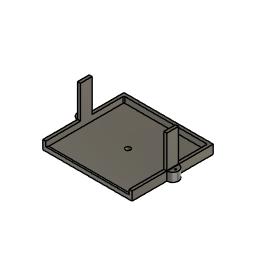
battery tray v7 (Autodesk Fusion 360 design; units mm, degrees)
Autodesk Fusion 360 part; units mm, degrees
sketch "Sketch1" plane through (0, 0, 0) normal (0, 0, 1) x (1, 0, 0)
  line L0 (0, 0) -> (0, 176.2125)
  line L1 (0, 176.2125) -> (193.675, 176.2125)
  line L2 (193.675, 176.2125) -> (193.675, 0)
  line L3 (193.675, 0) -> (0, 0)
  dimension "d21" = 193.675
  dimension "d22" = 176.2125
  constraint coincident L0.start L3.end
  constraint vertical L0
  constraint perpendicular L0 L1
  constraint perpendicular L1 L2
  constraint perpendicular L0 L3
  measures "d21" distance of L0 L2
  measures "d22" distance of L1 L3
extrude "Extrude1" add sketch "Sketch1" along normal blind 19.05
sketch "Sketch3" plane through (0, 0, 19.05) normal (0, 0, 1) x (-1, 0, 0)
  line L0 (-193.675, 0) -> (-193.675, -176.2125)
  line L1 (-193.675, -176.2125) -> (0, -176.2125)
  line L2 (0, -176.2125) -> (0, 0)
  line L3 (0, 0) -> (-193.675, 0)
  line L4 (-187.325, -6.35) -> (-6.35, -6.35)
  line L5 (-6.35, -6.35) -> (-6.35, -167.8305)
  line L6 (-8.382, -169.8625) -> (-185.293, -169.8625)
  line L7 (-187.325, -167.8305) -> (-187.325, -6.35)
  arc A0 (-187.325, -167.8305) -> (-185.293, -169.8625) centre (-185.293, -167.8305) ccw
  arc A1 (-8.382, -169.8625) -> (-6.35, -167.8305) centre (-8.382, -167.8305) ccw
  dimension "d13" = 180.975
  dimension "d14" = 163.5125
  dimension "d17" = 6.35
  dimension "d18" = 6.35
  dimension "d25" = 2.032
  dimension "d26" = 2.032
  constraint horizontal L4
  constraint vertical L5
  constraint horizontal L6
  constraint vertical L7
  constraint tangent L7 A0
  constraint tangent L6 A0
  constraint tangent L5 A1
  constraint tangent L6 A1
  constraint coincident L4.start L7.end
  constraint coincident L4.end L5.start
  measures "d13" distance of L5 L7
  measures "d14" distance of L4 L6
  measures "d17" distance of L3 L4
  measures "d18" distance of L2 L5
  measures "d25" radius of A0
  measures "d26" radius of A1
extrude "Extrude3" cut sketch "Sketch3" against normal blind 12.7 contours L4 L5 L6 L7 A0 A1
sketch "Sketch4" plane through (0, 0, 0) normal (0, 0, 1) x (1, 0, 0)
  line L0 (193.675, 176.2125) -> (193.675, 0)
  circle A0 centre (193.675, 88.1062) radius 12.7
  line L1 (193.675, 0) -> (0, 0)
  line L2 (0, 176.2125) -> (193.675, 176.2125)
  line L3 (0, 0) -> (0, 176.2125)
  circle A1 centre (0, 88.1062) radius 12.7
  dimension "d29" = 88.1063
  dimension "d30" = 88.1063
  dimension "d31" = 25.4
  dimension "d61" = 25.4
  constraint coincident L0 A0.centre
  measures "d29" distance of A0.centre L1
  measures "d30" distance of A0.centre L2
  measures "d31" diameter of A0
  measures "d61" diameter of A1
extrude "Extrude4" add sketch "Sketch4" along normal blind 19.05 contours L0 A0 | L3 A1 picked at (197.7369, 89.2989) picked at (-6.9833, 85.4668)
sketch "Sketch5" plane through (0, 0, 19.05) normal (0, 0, 1) x (-1, 0, 0)
  line L0 (-8.382, -169.8625) -> (-185.293, -169.8625)
  arc A0 (-187.325, -167.8305) -> (-185.293, -169.8625) centre (-185.293, -167.8305) ccw
  line L1 (-187.325, -167.8305) -> (-187.325, -6.35)
  line L2 (-187.325, -6.35) -> (-6.35, -6.35)
  line L3 (-6.35, -6.35) -> (-6.35, -167.8305)
  arc A1 (-8.382, -169.8625) -> (-6.35, -167.8305) centre (-8.382, -167.8305) ccw
  line L4 (-193.675, 0) -> (-193.675, -75.4062)
  arc A2 (-193.675, -75.4062) -> (-193.675, -100.8062) centre (-193.675, -88.1062) ccw
  line L5 (-193.675, -100.8062) -> (-193.675, -176.2125)
  line L6 (-193.675, -176.2125) -> (0, -176.2125)
  line L7 (0, -176.2125) -> (0, -100.8062)
  arc A3 (0, -100.8062) -> (0, -75.4062) centre (0, -88.1062) ccw
  line L8 (0, -75.4062) -> (0, 0)
  line L9 (0, 0) -> (-193.675, 0)
  circle A4 centre (-200.025, -88.1062) radius 1.651
  line L10 (-96.8375, 0) -> (-96.8375, -176.2125)
  circle A5 centre (6.35, -88.1062) radius 1.651
  line L11 (-193.675, 0) -> (0, 0)
  circle A6 centre (-193.675, -88.1062) radius 12.7
  line L12 (0, -88.1062) -> (-193.675, -88.1062)
  point P0 (-193.675, -88.1062)
  dimension "d35" = 3.302
  dimension "d37" = 6.35
  dimension "d38" = 88.1063
  dimension "d39" = 25.4
  constraint symmetric A4 L10 A5
  constraint coincident A3.centre L12.start
  constraint coincident P0 A2.centre
  measures "d35" diameter of A4
  measures "d37" distance of A4.centre P0
  measures "d38" distance of A4.centre L11
  measures "d39" diameter of A6
sketch "Sketch7" plane through (0, 0, 0) normal (0, 0, 1) x (1, 0, 0)
  circle A0 centre (96.8375, 88.1063) radius 1.651
  dimension "d42" = 3.302
  measures "d42" diameter of A0
sketch "Sketch8" plane through (0, 0, 19.05) normal (0, 0, 1) x (-1, 0, 0)
  line L0 (-8.382, -169.8625) -> (-185.293, -169.8625)
  arc A0 (-187.325, -167.8305) -> (-185.293, -169.8625) centre (-185.293, -167.8305) ccw
  line L1 (-187.325, -167.8305) -> (-187.325, -6.35)
  line L2 (-187.325, -6.35) -> (-6.35, -6.35)
  line L3 (-6.35, -6.35) -> (-6.35, -167.8305)
  arc A1 (-8.382, -169.8625) -> (-6.35, -167.8305) centre (-8.382, -167.8305) ccw
  line L4 (-193.675, 0) -> (-193.675, -75.4062)
  arc A2 (-193.675, -75.4062) -> (-193.675, -100.8062) centre (-193.675, -88.1062) ccw
  line L5 (-193.675, -100.8062) -> (-193.675, -176.2125)
  line L6 (-193.675, -176.2125) -> (0, -176.2125)
  line L7 (0, -176.2125) -> (0, -100.8062)
  arc A3 (0, -100.8062) -> (0, -75.4062) centre (0, -88.1062) ccw
  line L8 (0, -75.4062) -> (0, 0)
  line L9 (0, 0) -> (-193.675, 0)
  circle A4 centre (6.35, -88.1062) radius 1.651
  line L10 (-6.35, -6.35) -> (-6.35, -167.8305)
  line L11 (-96.8375, 0) -> (-96.8375, -176.2125)
  circle A5 centre (-200.025, -88.1062) radius 1.651
  line L12 (0, 0) -> (0, -176.2125)
  dimension "d48" = 3.302
  dimension "d49" = 6.35
  constraint midpoint L9 L11.start
  constraint midpoint L6 L11.end
  constraint symmetric A4 L11 A5
  measures "d48" diameter of A5
  measures "d49" distance of A4.centre L12
extrude "Extrude5" cut sketch "Sketch8" against normal blind 19.05 contours A4 | A5
extrude "Extrude6" cut sketch "Sketch7" along normal blind 6.35 draft 30
sketch "Sketch9" plane through (0, 0, 19.05) normal (0, 0, 1) x (-1, 0, 0)
  line L0 (0, -100.8062) -> (-6.35, -100.8062)
  line L1 (-6.35, -100.8062) -> (-6.35, -75.4062)
  line L2 (-6.35, -75.4062) -> (0, -75.4062)
  line L3 (0, -75.4062) -> (0, -100.8062)
  line L4 (-96.8375, 0) -> (-96.8375, -176.2125)
  line L5 (-187.325, -75.4062) -> (-193.675, -75.4062)
  line L6 (-193.675, -75.4062) -> (-193.675, -100.8062)
  line L7 (-187.325, -100.8062) -> (-187.325, -75.4062)
  line L8 (-193.675, -100.8062) -> (-187.325, -100.8062)
  point P0 (0, -75.4062)
  point P1 (0, -100.8062)
  dimension "d62" = 6.35
  constraint horizontal L0
  constraint perpendicular L0 L1
  constraint perpendicular L1 L2
  constraint perpendicular L0 L3
  constraint coincident P0 L2.end
  constraint coincident L0.start L3.end
  constraint symmetric L0.start L4 L6.end
  constraint symmetric L0.end L4 L7.start
  constraint symmetric L1.end L4 L5.start
  constraint symmetric P0 L4 L5.end
  measures "d62" distance of L1 L3
extrude "Extrude7" add sketch "Sketch9" along normal blind 71.12
fillet "Fillet1" radius 0.635 1 edges at (193.675, 88.1062, 19.05)
fillet "Fillet2" radius 0.635 1 edges at (0, 88.1062, 19.05)
sketch "Sketch10" plane through (0, 0, 19.05) normal (0, 0, 1) x (-1, 0, 0)
  line L0 (-193.675, -75.4062) -> (-187.325, -75.4062)
  line L1 (-187.325, -75.4062) -> (-187.325, -6.35)
  line L2 (-187.325, -6.35) -> (-6.35, -6.35)
  line L3 (-6.35, -6.35) -> (-6.35, -75.4062)
  line L4 (-6.35, -75.4062) -> (0, -75.4062)
  line L5 (0, -75.4062) -> (0, 0)
  line L6 (0, 0) -> (-193.675, 0)
  line L7 (-193.675, 0) -> (-193.675, -75.4062)
  line L8 (-6.35, -6.35) -> (-6.35, 0)
  line L9 (-6.35, 0) -> (-187.452, 0)
  line L10 (-187.325, -6.35) -> (-187.325, 0)
  line L11 (-187.325, -6.35) -> (-6.35, -6.35)
  constraint coincident L2.end L3.start
  constraint coincident L6 L8.end
  constraint perpendicular L6 L8
  constraint coincident L6 L9.end
  constraint coincident L1.end L2.start
  constraint coincident L6 L10.end
extrude "Extrude8" cut sketch "Sketch10" against normal blind 10.16 contours L2 L6 L8 L9 L10 L11
sketch "Sketch12" plane through (193.675, 0, 0) normal (1, 0, 0) x (0, 1, 0)
  line L0 (75.4062, 0) -> (75.4062, 19.05)
  line L1 (75.4062, 19.05) -> (0, 19.05)
  line L2 (0, 19.05) -> (0, 0)
  line L3 (0, 0) -> (75.4062, 0)
  line L4 (6.35, 6.35) -> (0, 8.89)
  line L5 (6.35, 6.35) -> (6.35, 8.89)
  line L6 (6.35, 8.89) -> (0, 8.89)
  constraint coincident L2 L4.end
  constraint vertical L5
  constraint perpendicular L2 L6
extrude "Extrude9" cut sketch "Sketch12" against normal up to surface (180.975 mm away) from surface at -6.35 contours L4 L5 L6
equation "d13 = 7 1/8\""
equation "d14 = 6 7/16\""
equation "d21 = d13 + 0.5 in"
equation "d22 = d14 + 0.5 in"
equation "d29 = d30"
equation "d30 = 0.5 * d22"
equation "d37 = 0.25 * d39"
equation "d38 = 0.5 * d22"
equation "d61 = d31"
